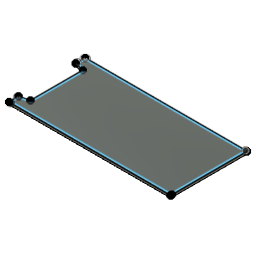
coolingpadbox v9 - Copy (Autodesk Fusion 360 design; units mm, degrees)
Autodesk Fusion 360 part; units mm, degrees
sketch "Sketch1" plane through (0, 0, 0) normal (1, 0, 0) x (0, 1, 0)
sketch "Sketch2" plane through (0, 0, 0) normal (0, 1, 0) x (1, 0, 0)
sketch "Sketch3" plane through (0, 0, 0) normal (0, 0, 1) x (1, 0, 0)
  line L0 (-89.6492, -40) -> (80, -40)
  line L1 (80, -40) -> (80, 40)
  line L2 (80, 40) -> (-89.6492, 40)
  line L3 (-89.6492, 40) -> (-89.6492, 30)
  line L4 (-89.6492, -40) -> (-89.6492, -30)
  line L5 (-89.6492, -40) -> (-79.6492, -40)
  line L6 (-79.6492, 27.5) -> (-79.6492, -27.5)
  line L7 (-79.6492, 27.5) -> (-89.6492, 30)
  line L8 (-89.6492, -30) -> (-79.6492, -27.5)
  constraint horizontal L0
  constraint perpendicular L0 L1
  constraint perpendicular L1 L2
  constraint coincident L0 L5.end
extrude "Extrude1" add sketch "Sketch3" along normal blind 2.5
sketch "Sketch4" plane through (0, 0, 2.5) normal (0, 0, 1) x (-1, 0, 0)
  line L0 (89.6492, 40) -> (-80, 40)
  line L1 (-80, 40) -> (-80, -40)
  line L2 (-80, -40) -> (89.6492, -40)
  line L3 (89.6492, -40) -> (89.6492, -30)
  line L4 (89.6492, -30) -> (79.6492, -27.5)
  line L5 (79.6492, -27.5) -> (79.6492, 27.5)
  line L6 (79.6492, 27.5) -> (89.6492, 30)
  line L7 (89.6492, 30) -> (89.6492, 40)
  line L8 (89.6492, -40) -> (-80, -40)
  line L9 (-80, -40) -> (-80, 40)
  line L10 (89.6492, 40) -> (-80, 40)
  line L11 (89.6492, 30) -> (89.6492, 40)
  line L12 (89.6492, 30) -> (79.6492, 27.5)
  line L13 (79.6492, 27.5) -> (79.6492, -27.5)
  line L14 (79.6492, -27.5) -> (89.6492, -30)
  line L15 (89.6492, -40) -> (89.6492, -30)
  line L16 (89.6492, -40) -> (89.6492, -38.5)
  line L17 (88.1492, -38.5) -> (-78.5, -38.5)
  line L18 (-80, -40) -> (-78.5, -40)
  line L19 (-78.5, -38.5) -> (-78.5, 38.5)
  line L20 (-80, 40) -> (-80, 38.5)
  line L21 (-78.5, 38.5) -> (88.1492, 38.5)
  line L22 (89.6492, 40) -> (88.1492, 40)
  line L23 (88.1492, 38.5) -> (88.1492, 31)
  line L24 (89.6492, 30) -> (89.6492, 31.375)
  line L25 (88.1492, 31) -> (78.1492, 28.5)
  line L26 (78.1492, -28.4841) -> (78.1492, 28.5)
  line L27 (89.6492, -40) -> (88.1492, -40)
  line L28 (88.1492, -31.1066) -> (88.1492, -38.5)
  line L29 (89.6492, -30) -> (89.6492, -31.5)
  line L30 (88.1492, -31.1066) -> (78.1492, -28.4841)
  dimension "d9" = 1.5
  dimension "d11" = 1.5
  constraint coincident L2.end L3.start
  constraint coincident L1.end L2.start
  constraint coincident L0.end L1.start
  constraint coincident L0.start L7.end
  constraint coincident L6.end L7.start
  constraint coincident L5.end L6.start
  constraint coincident L4.end L5.start
  constraint coincident L3.end L4.start
  constraint coincident L15 L16.end
  constraint perpendicular L1 L17
  constraint coincident L2 L18.end
  constraint perpendicular L9 L18
  constraint perpendicular L0 L19
  constraint coincident L1 L20.end
  constraint coincident L10 L22.end
  constraint perpendicular L0 L23
  constraint coincident L11 L24.end
  constraint parallel L6 L25
  constraint coincident L8 L27.end
  constraint perpendicular L2 L28
  constraint coincident L15 L29.end
  measures "d9" distance of L0.end L20.end
  measures "d11" distance of L0.start L22.end
